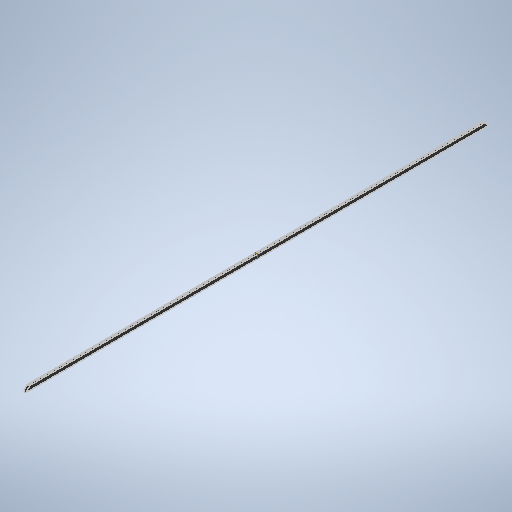
# Autodesk Inventor part: JUNTA DE GOMA 800MM
Saved by Autodesk Inventor 2025 (Build 290162000, 162)
## iProperties
Created: 2026-02-11
Part Number: JUNTA DE GOMA 800MM
Material: Rubber
Document SubType Name: Modeling
Designer: Frank
Density: 0.93 g/cm^3
Appearance: Rubber - Black
Author: Frank
Autodesk Inventor part; units mm, degrees
ref_plane "YZ Plane" through (0, 0, 0) normal (1, 0, 0) x (0, 1, 0)
ref_plane "XZ Plane" through (0, 0, 0) normal (0, 1, 0) x (-1, 0, 0)
ref_plane "XY Plane" through (0, 0, 0) normal (0, 0, 1) x (1, 0, 0)
sketch "Sketch1" plane through (0, 0, 0) normal (0, 0, 1) x (1, 0, 0)
  line L0 (-8.5, 42.6) -> (-6.1, 42.6)
  line L1 (-6.1, 36.1) -> (-8.5, 36.1)
  line L2 (-6.1, 36.1) -> (-6.1, 42.6)
  line L3 (-8.5, 37.35) -> (-8.5, 36.1)
  line L4 (-8.5, 41.35) -> (-8.5, 42.6)
  line L5 (-8.5, 37.35) -> (-9.2058, 37.35)
  line L6 (-8.5, 41.35) -> (-9.2058, 41.35)
  line L7 (-9.9, 42.36) -> (-9.2058, 41.35)
  line L8 (-9.9, 36.34) -> (-9.2058, 37.35)
  line L9 (-9.9, 42.36) -> (-9.9, 36.34)
  point P0 (-8.5, 41.975)
  point P1 (-6.1, 39.35)
  dimension "d27" = 6.5
  dimension "d28" = 2.4
  dimension "d29" = 2.4
  dimension "d35" = 111
  dimension "d36" = 4
  dimension "d37" = 6.02
  dimension "d38" = 0.7058
  dimension "d39" = 0.7058
  dimension "d43" = 3.01
  dimension "d44" = 2
  constraints: 20 end point, 3 horizontal, 2 midpoint, 2 perpendicular, 1 equal length
  measures "d27" distance between parallel lines of L1 L0
  measures "d28" distance from line of L0.start L2
  measures "d29" distance of L1.start L1.end
  measures "d35" angle of L8 L7
  measures "d36" distance between parallel lines of L5 L6
  measures "d37" distance of L8.start L7.start
  measures "d38" distance of L4.start L6.end
  measures "d39" distance of L3.start L5.end
  measures "d43" vertical distance of point (-6.1, 39.35) L7.start
  measures "d44" distance from line of point (-6.1, 39.35) L6
extrude "Extrusion1" add sketch "Sketch1" against normal blind 727.8
ref_plane "Plano de trabajo3" through (0, 0, -363.9) normal (0, 0, 1) x (1, 0, 0)
sketch "Boceto2" plane through (-6.1, 36.1, 0) normal (1, 0, 0) x (0, 0, -1)
  line L0 (0, 0) -> (6.5, 6.5)
  line L1 (0, 6.5) -> (727.8, 6.5) projected
  line L2 (6.5, 6.5) -> (0, 6.5)
  line L3 (0, 0) -> (0, 6.5)
  line L4 (0, 6.26) -> (0, 0.24) projected
  point P0 (0, -36.1)
  dimension "d60" = 45
  constraints: 6 end point, 2 collinear, 1 point on line
  measures "d60" angle of L3 L0
extrude "Extrusión2" cut sketch "Boceto2" against normal through all
mirror "Simetría2" about plane through (0, 0, -363.9) normal (0, 0, 1) of "Extrusión2"
body "Solid1"
